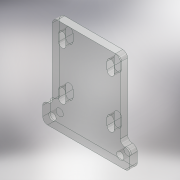
# Autodesk Inventor part: SecondaryEncoderPCBMount
Saved by Autodesk Inventor 2018.2 (Build 222227000, 227)
## iProperties
Created: 2018-03-28
Part Number: SecondaryEncoderPCBMount
Material: ABS Plastic
Document SubType Name: Modeling
Designer: Muchen He
Density: 1.06 g/cm^3
Appearance: Clear
Author: Muchen He
Autodesk Inventor part; units mm, degrees
ref_plane "YZ Plane" through (0, 0, 0) normal (1, 0, 0) x (0, 1, 0)
ref_plane "XZ Plane" through (0, 0, 0) normal (0, 1, 0) x (-1, 0, 0)
ref_plane "XY Plane" through (0, 0, 0) normal (0, 0, 1) x (1, 0, 0)
sketch "Sketch1" plane through (0, 0, 0) normal (0, 1, 0) x (-1, 0, 0)
  line L0 (10, -10) -> (-10, -10) construction
  line L1 (-10, -10) -> (-10, 10) construction
  line L2 (-10, 10) -> (10, 10) construction
  line L3 (10, 10) -> (10, -10) construction
  line L4 (10, -10) -> (-10, 10) construction
  line L5 (-10, -10) -> (10, 10) construction
  line L6 (10, -10) -> (10, -7) construction
  line L7 (11.5, -10) -> (11.5, -7)
  line L8 (8.5, -7) -> (8.5, -10)
  arc A0 (8.5, -10) -> (11.5, -10) centre (10, -10) ccw
  arc A1 (11.5, -7) -> (8.5, -7) centre (10, -7) ccw
  line L9 (-10, -10) -> (-10, -7) construction
  line L10 (-8.5, -10) -> (-8.5, -7)
  line L11 (-11.5, -7) -> (-11.5, -10)
  arc A2 (-11.5, -10) -> (-8.5, -10) centre (-10, -10) ccw
  arc A3 (-8.5, -7) -> (-11.5, -7) centre (-10, -7) ccw
  line L12 (10, 10) -> (10, 13) construction
  line L13 (11.5, 10) -> (11.5, 13)
  line L14 (8.5, 13) -> (8.5, 10)
  arc A4 (8.5, 10) -> (11.5, 10) centre (10, 10) ccw
  arc A5 (11.5, 13) -> (8.5, 13) centre (10, 13) ccw
  line L15 (-10, 10) -> (-10, 13) construction
  line L16 (-8.5, 10) -> (-8.5, 13)
  line L17 (-11.5, 13) -> (-11.5, 10)
  arc A6 (-11.5, 10) -> (-8.5, 10) centre (-10, 10) ccw
  arc A7 (-8.5, 13) -> (-11.5, 13) centre (-10, 13) ccw
  circle A8 centre (14, -18) radius 1.5
  circle A9 centre (-14, -18) radius 1.5
  line L18 (14, -18) -> (-14, -18) construction
  line L19 (18, -22) -> (-18, -22)
  line L20 (-18, -22) -> (-18, -14)
  line L21 (-18, -14) -> (-14, -14)
  line L22 (-14, -14) -> (-14, 17.5)
  line L23 (-14, 17.5) -> (14, 17.5)
  line L24 (14, 17.5) -> (14, -14)
  line L25 (14, -14) -> (18, -14)
  line L26 (18, -14) -> (18, -22)
  point P0 (0, 0)
  point P1 (10, -8.5)
  point P2 (-10, -8.5)
  point P3 (10, 11.5)
  point P4 (-10, 11.5)
  point P5 (0, -18)
  point P6 (0, 0)
  point P7 (0, -22)
  dimension "d0" = 20
  dimension "d1" = 20
  dimension "d2" = 3
  dimension "d3" = 3
  dimension "d4" = 3
  dimension "d5" = 3
  dimension "d6" = 3
  dimension "d7" = 3
  dimension "d8" = 3
  dimension "d9" = 3
  dimension "d10" = 3
  dimension "d11" = 8
  dimension "d12" = 28
  dimension "d13" = 4
  dimension "d15" = 4
  dimension "d16" = 4
  dimension "d17" = 36
  dimension "d18" = 3
  constraints: 62 end point, 16 point on circle, 16 tangent, 10 centre point, 9 midpoint, 7 perpendicular, 6 parallel, 3 horizontal, 3 point on line, 2 equal length, 2 vertical, 2 vertical alignment, 1 equal radius
  measures "d0" distance of L1.end L2.end
  measures "d1" distance of L0.end L1.end
  measures "d2" distance of L0.start L6.end
  measures "d3" diameter of A1
  measures "d4" distance of L0.end L9.end
  measures "d5" diameter of A3
  measures "d6" distance of L2.end L12.end
  measures "d7" diameter of A5
  measures "d8" distance of L1.end L15.end
  measures "d9" diameter of A7
  measures "d10" diameter of A9
  measures "d11" distance between parallel lines of L0 L18
  measures "d12" distance of L18.start L18.end
  measures "d13" distance between parallel lines of L18 L19
  measures "d15" distance between parallel lines of L1 L22
  measures "d16" distance between parallel lines of L18 L21
  measures "d17" distance of L19.start L19.end
  measures "d18" distance edge to line of A7 L23
extrude "Extrusion1" add sketch "Sketch1" along normal blind 3
fillet "Fillet1" radius 2 8 edges at (14, 1.5, -14) (14, 1.5, 17.5) (-14, 1.5, 17.5) (-14, 1.5, -14) (-18, 1.5, -14) (-18, 1.5, -22) (18, 1.5, -22) (18, 1.5, -14)
body "Solid1"
